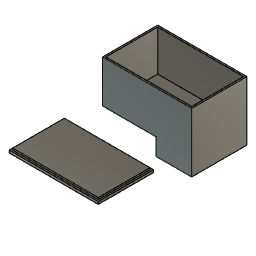
PULT AND KRISHKA (Autodesk Fusion 360 design; units mm, degrees)
Autodesk Fusion 360 part; units mm, degrees
note: some values were not read from the file. Set by a fixed rule: which face or edge a step refers to.
sketch "Sketch1" plane through (0, 0, 0) normal (0, 0, 1) x (1, 0, 0)
  line L0 (-50, 50) -> (55, 50)
  line L1 (55, 50) -> (55, -15)
  line L2 (55, -15) -> (-50, -15)
  line L3 (-50, -15) -> (-50, 50)
  dimension "d1" = 105
  dimension "d2" = 65
  constraint horizontal L0
  constraint vertical L1
  constraint horizontal L2
  constraint vertical L3
  measures "d1" distance of L0.start L0.end
  measures "d2" distance of L0.start L2.end
extrude "Extrude1" add sketch "Sketch1" along normal blind 50 makes body 1
shell "Shell1" thickness 2 removed faces 1 at (-15, 28.3333, 50) on bodies 1
sketch "Sketch2" plane through (0, 0, 0) normal (0, 0, 1) x (1, 0, 0)
  line L0 (-50, -25) -> (55, -25)
  line L1 (55, -25) -> (55, -90)
  line L2 (55, -90) -> (-50, -90)
  line L3 (-50, -90) -> (-50, -25)
  dimension "d6" = 105
  dimension "d7" = 65
  constraint horizontal L0
  constraint vertical L1
  constraint horizontal L2
  constraint vertical L3
  measures "d6" distance of L0.start L0.end
  measures "d7" distance of L0.start L2.end
extrude "Extrude2" add sketch "Sketch2" along normal blind 3 separate body makes body 2
shell "Shell2" thickness 2 removed faces 1 at (-15, -46.6667, 3) on bodies 2
extrude "Extrude3" add 1 faces at (-14.3333, -67.6667, 2) along direction (0, 0, 1) blind 3 on bodies 2 bodies 2
sketch "Sketch3" plane through (0, 0, 0) normal (0, 0, 1) x (1, 0, 0)
  line L0 (55, -15) -> (13, -15)
  line L1 (13, -15) -> (13, 50)
  line L2 (13, 50) -> (55, 50)
  line L3 (55, 50) -> (55, -15)
  dimension "d13" = 42
  dimension "d14" = 65
  constraint horizontal L0
  constraint vertical L1
  constraint horizontal L2
  constraint vertical L3
  measures "d13" distance of L0.start L0.end
  measures "d14" distance of L0.start L2.end
extrude "Extrude4" add sketch "Sketch3" against normal blind 20 bodies 1
sketch "Sketch4" plane through (0, 50, 0) normal (0, 1, 0) x (-1, 0, 0)
  line L0 (-13, 0) -> (50, 0)
  line L1 (50, 0) -> (50, 50)
  line L2 (50, 50) -> (-55, 50)
  line L3 (-55, 50) -> (-55, -20)
  line L4 (-55, -20) -> (-13, -20)
  line L5 (-13, -20) -> (-13, 0)
  line L6 (-13, -20) -> (-13, -18)
  line L7 (-55, -20) -> (-53, -20)
  line L8 (-13, 0) -> (-13, -2)
  line L9 (-13, -2) -> (-55, -2)
  line L10 (-13, -18) -> (-55, -18)
  line L11 (-53, -20) -> (-53, 2.2415)
  line L12 (-13, -20) -> (-15, -20)
  line L13 (-15, -20) -> (-15, 0.4719)
  dimension "d17" = 2
  dimension "d18" = 2
  dimension "d19" = 2
  dimension "d20" = 2
  constraint coincident L4.end L5.start
  constraint perpendicular L4 L6
  constraint coincident L3.end L4.start
  constraint perpendicular L3 L7
  constraint coincident L0.start L5.end
  constraint perpendicular L0 L8
  constraint coincident L3 L9.end
  constraint perpendicular L3 L9
  constraint coincident L3 L10.end
  constraint perpendicular L3 L10
  constraint perpendicular L9 L11
  constraint perpendicular L5 L12
  constraint perpendicular L9 L13
  measures "d17" distance of L4.end L6.end
  measures "d18" distance of L3.end L7.end
  measures "d19" distance of L0.start L8.end
  measures "d20" distance of L4.end L12.end
extrude "Extrude5" cut sketch "Sketch4" against normal blind 63 contours L9 L10 L11 L13 bodies 1
sketch "Sketch5" plane through (0, -15, 0) normal (0, -1, 0) x (1, 0, 0)
  line L0 (55, -20) -> (55, 50)
  line L1 (55, 50) -> (-50, 50)
  line L2 (-50, 50) -> (-50, 0)
  line L3 (-50, 0) -> (13, 0)
  line L4 (13, 0) -> (13, -20)
  line L5 (13, -20) -> (55, -20)
move_body "Move1" bodies 2 to x (1, 0, 0) y (0, -1, 0) z (0, 0, -1) at (0, -40, 57)
move_body "Move2" bodies 2 to x (1, 0, 0) y (0, -1, 0) z (0, 0, -1) at (0, -135, 104)
move_body "Move3" bodies 2 to x (1, 0, 0) y (0, 1, 0) z (0, 0, 1) at (0, 60, -40)
